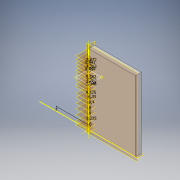
# Autodesk Inventor part: 2nd try
Saved by Autodesk Inventor 2018 (Build 220112000, 112)
## iProperties
Created: 2020-05-21
Part Number: 2nd try
Material: Generic
Document SubType Name: Modeling
Designer: natha
Density: 1 g/cm^3
Appearance: Default
Author: natha
Autodesk Inventor part; units mm, degrees
sketch "Sketch1" plane through (0, 0, 0) normal (0, 0, 1) x (1, 0, 0)
  line L0 (0, 0) -> (80, 0)
  line L1 (80, 0) -> (80, 120)
  line L2 (80, 120) -> (0, 120)
  line L3 (0, 120) -> (0, 0)
  line L4 (-16, 0) -> (96, 0) projected
  line L5 (0, 144) -> (0, -24) projected
  dimension "d0" = 120
  dimension "d1" = 80
  constraints: 8 end point, 2 parallel, 1 horizontal, 1 perpendicular
  measures "d0" distance between parallel lines of L4 L2
  measures "d1" distance between parallel lines of L5 L1
extrude "Extrusion1" add sketch "Sketch1" against normal blind 10
ref_plane "Waste_Output_y" through (0, 10, 0) normal (0, 1, 0) x (-1, 0, 0)
ref_plane "lower_vial_2_vial_y" through (0, 15, 0) normal (0, 1, 0) x (-1, 0, 0)
ref_plane "mux_valves_4" through (0, 60, 0) normal (0, 1, 0) x (-1, 0, 0)
ref_plane "mux_valves_3" through (0, 50, 0) normal (0, 1, 0) x (-1, 0, 0)
sketch "y_coordinates" plane through (0, 0, 0) normal (0, 0, 1) x (1, 0, 0)
  line L0 (0, 0) -> (0, 120) projected
  line L1 (-84, 0) -> (84, 0) projected
  point P0 (0, 7)
  point P1 (0, 13)
  point P2 (0, 22.225)
  point P3 (0, 31.225)
  point P4 (0, 39.225)
  point P5 (0, 47.625)
  point P6 (0, 53.975)
  point P7 (0, 63.5)
  point P8 (0, 67.5789)
  point P9 (0, 73.025)
  point P10 (0, 77.7875)
  point P11 (0, 83.3695)
  point P12 (0, 87.8661)
  point P13 (0, 93.6625)
  point P14 (0, 98.425)
  point P15 (0, 103.8658)
  point P16 (0, 109.5375)
  dimension "d11" = 7
  dimension "d12" = 6
  dimension "d13" = 9.225
  dimension "d14" = 9
  dimension "d15" = 8
  dimension "d16" = 8.4
  dimension "d17" = 6.35
  dimension "d18" = 9.525
  dimension "d19" = 4.0789
  dimension "d20" = 5.4461
  dimension "d21" = 4.7625
  dimension "d22" = 5.582
  dimension "d23" = 4.4966
  dimension "d24" = 5.7964
  dimension "d25" = 4.7625
  dimension "d26" = 5.4408
  dimension "d27" = 5.6717
  constraints: 18 other
  measures "d11" distance from line of point (0, 7) L1
  measures "d12" distance of point (0, 7) point (0, 13)
  measures "d13" distance of point (0, 13) point (0, 22.225)
  measures "d14" distance of point (0, 22.225) point (0, 31.225)
  measures "d15" distance of point (0, 31.225) point (0, 39.225)
  measures "d16" distance of point (0, 39.225) point (0, 47.625)
  measures "d17" distance of point (0, 53.975) point (0, 47.625)
  measures "d18" distance of point (0, 63.5) point (0, 53.975)
  measures "d19" distance of point (0, 67.579) point (0, 63.5)
  measures "d20" distance of point (0, 73.025) point (0, 67.579)
  measures "d21" distance of point (0, 73.025) point (0, 77.788)
  measures "d22" distance of point (0, 83.369) point (0, 77.788)
  measures "d23" distance of point (0, 87.866) point (0, 83.369)
  measures "d24" distance of point (0, 93.662) point (0, 87.866)
  measures "d25" distance of point (0, 98.425) point (0, 93.662)
  measures "d26" distance of point (0, 103.866) point (0, 98.425)
  measures "d27" distance of point (0, 109.537) point (0, 103.866)
ref_plane "y_waste_output" through (0, 7, 0) normal (0, 1, 0) x (-1, 0, 0)
ref_plane "y_lower_vial_2_vial" through (0, 13, 0) normal (0, 1, 0) x (-1, 0, 0)
ref_plane "y_lower_mux" through (0, 22.225, 0) normal (0, 1, 0) x (-1, 0, 0)
ref_plane "y_mux_valves_1" through (0, 31.225, 0) normal (0, 1, 0) x (-1, 0, 0)
ref_plane "y_mux_valves_2" through (0, 39.225, 0) normal (0, 1, 0) x (-1, 0, 0)
ref_plane "y_mux_valves_3" through (0, 47.625, 0) normal (0, 1, 0) x (-1, 0, 0)
ref_plane "y_mux_valves_4" through (0, 53.975, 0) normal (0, 1, 0) x (-1, 0, 0)
ref_plane "y_from_vial" through (0, 63.5, 0) normal (0, 1, 0) x (-1, 0, 0)
ref_plane "y_from_vial_valves" through (0, 67.5789, 0) normal (0, 1, 0) x (-1, 0, 0)
ref_plane "y_from_vial_line" through (0, 73.025, 0) normal (0, 1, 0) x (-1, 0, 0)
ref_plane "y_bypass_valves" through (0, 77.7875, 0) normal (0, 1, 0) x (-1, 0, 0)
ref_plane "y_to_vial_line" through (0, 83.3695, 0) normal (0, 1, 0) x (-1, 0, 0)
ref_plane "y_to_vial_valves" through (0, 87.8661, 0) normal (0, 1, 0) x (-1, 0, 0)
ref_plane "y_to_vial" through (0, 93.6625, 0) normal (0, 1, 0) x (-1, 0, 0)
ref_plane "y_demux_valves_1" through (0, 98.425, 0) normal (0, 1, 0) x (-1, 0, 0)
ref_plane "y_demux_valves_2" through (0, 103.8658, 0) normal (0, 1, 0) x (-1, 0, 0)
ref_plane "y_demux_valves_3" through (0, 109.5375, 0) normal (0, 1, 0) x (-1, 0, 0)
ref_plane "lower_mux_y" through (0, 20, 0) normal (0, 1, 0) x (-1, 0, 0)
ref_plane "mux_valves_1" through (0, 30, 0) normal (0, 1, 0) x (-1, 0, 0)
ref_plane "mux_valves_2" through (0, 40, 0) normal (0, 1, 0) x (-1, 0, 0)
body "Solid1"
